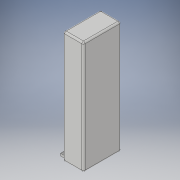
# Autodesk Inventor part: Аккумулятор
Saved by Autodesk Inventor 2019 (Build 230136000, 136)
## iProperties
Created: 2020-10-19
Part Number: Аккумулятор
Material: Типовые
Document SubType Name: Modeling
Designer: Surflay
Density: 1 g/cm^3
Appearance: По умолчанию
Author: Surflay
Autodesk Inventor part; units mm, degrees
ref_plane "YZ Plane" through (0, 0, 0) normal (1, 0, 0) x (0, 1, 0)
ref_plane "XZ Plane" through (0, 0, 0) normal (0, 1, 0) x (-1, 0, 0)
ref_plane "XY Plane" through (0, 0, 0) normal (0, 0, 1) x (1, 0, 0)
sketch "Эскиз1" plane through (0, 0, 0) normal (0, 1, 0) x (-1, 0, 0)
  line L0 (180.5057, 0) -> (155.5057, 0)
  line L1 (155.5057, 0) -> (155.5057, -46)
  line L2 (155.5057, -46) -> (180.5057, -46)
  line L3 (180.5057, -46) -> (180.5057, 0)
  point P0 (0, 0)
  dimension "d0" = 25
  dimension "d1" = 46
  constraints: 8 end point, 2 parallel, 1 horizontal, 1 perpendicular
  measures "d0" distance of L2.end L1.end
  measures "d1" distance of L1.end L0.end
extrude "Выдавливание1" add sketch "Эскиз1" along normal blind 138
fillet "Сопряжение1" radius 2 12 edges at (-155.5057, 69, 0) (-155.5057, 69, -46) (-155.5057, 138, -23) (-155.5057, 0, -23) (-168.0057, 138, 0) (-168.0057, 138, -46) (-180.5057, 138, -23) (-180.5057, 69, 0) (-180.5057, 69, -46) (-180.5057, 0, -23) (-168.0057, 0, 0) (-168.0057, 0, -46)
sketch "Эскиз2" plane through (-180.5057, 2, -2) normal (-1, 0, 0) x (0, 0, 1)
  line L0 (-42.0719, 0.0612) -> (-37.0719, 0.0612)
  line L1 (-37.0719, 0.0612) -> (-37.0719, 3.0612)
  line L2 (-37.0719, 3.0612) -> (-42.0719, 3.0612)
  line L3 (-42.0719, 3.0612) -> (-42.0719, 0.0612)
  line L4 (0, 0) -> (-42, 0) projected
  line L5 (0, 0) -> (-5, 0)
  line L6 (-5, 0) -> (-5, 3)
  line L7 (-5, 3) -> (0, 3)
  line L8 (0, 3) -> (0, 0)
  point P0 (2, -2)
  dimension "d5" = 5
  dimension "d6" = 3
  dimension "d7" = 5
  dimension "d8" = 3
  constraints: 16 end point, 4 parallel, 2 horizontal, 2 perpendicular
  measures "d5" distance of L2.end L1.end
  measures "d6" distance of L1.end L0.end
  measures "d7" distance of L6.end L7.end
  measures "d8" distance of L5.end L6.end
extrude "Выдавливание2" add sketch "Эскиз2" along normal blind 5
